Autodesk Fusion 360 part; units mm, degrees
(part 3 of 5)
  line L423 (12.6531, -24.0922) -> (12.4457, -24.1094)
  line L424 (12.4457, -24.1094) -> (12.4457, -24.8166)
  line L425 (12.4457, -24.8166) -> (12.4457, -25.5237)
  line L426 (12.4457, -25.5237) -> (12.7147, -25.4972)
  spline S462 degree 3 poles (12.7147, -25.4972) (13.8566, -25.3848) (14.5858, -24.55) (14.5858, -23.3547) knots 0 0 0 0 1 1 1 1
  spline S463 degree 3 poles (14.5858, -23.3547) (14.5858, -21.5094) (12.6861, -20.5298) (11.4358, -21.7302) knots 0 0 0 0 1 1 1 1
  spline S464 degree 3 poles (11.4358, -21.7302) (11.2215, -21.9362) (11.1899, -21.9548) (11.1445, -21.9001) knots 0 0 0 0 1 1 1 1
  spline S465 degree 3 poles (11.1445, -21.9001) (10.8088, -21.4956) (9.9864, -21.3436) (9.4539, -21.5878) knots 0 0 0 0 1 1 1 1
  spline S466 degree 3 poles (9.4539, -21.5878) (8.7681, -21.9022) (8.3471, -22.7631) (8.4716, -23.5972) knots 0 0 0 0 1 1 1 1
  spline S467 degree 3 poles (8.8609, -38.3358) (9.1911, -37.3218) (10.383, -36.7997) (11.3154, -37.2606) knots 0 0 0 0 1 1 1 1
  spline S468 degree 3 poles (11.3154, -37.2606) (11.5789, -37.391) (11.712, -37.5031) (12.4391, -38.2065) knots 0 0 0 0 1 1 1 1
  spline S469 degree 3 poles (12.4391, -38.2065) (13.0246, -38.7727) (13.2898, -39.0048) (13.352, -39.0048) knots 0 0 0 0 1 1 1 1
  line L427 (13.352, -39.0048) -> (13.4394, -39.0048)
  line L428 (13.4394, -39.0048) -> (13.4394, -38.0493)
  line L429 (13.4394, -38.0493) -> (13.4394, -37.0938)
  line L430 (13.4394, -37.0938) -> (13.7641, -37.0938)
  line L431 (13.7641, -37.0938) -> (14.0891, -37.0938)
  line L432 (14.0891, -37.0938) -> (14.0888, -38.957)
  line L433 (14.0888, -38.957) -> (14.0888, -40.8199)
  line L434 (14.0888, -40.8199) -> (13.1993, -39.9218)
  spline S470 degree 3 poles (13.1993, -39.9218) (12.7098, -39.4279) (12.0642, -38.7689) (11.7643, -38.4573) knots 0 0 0 0 1 1 1 1
  spline S471 degree 3 poles (11.7643, -38.4573) (11.0509, -37.7164) (10.6839, -37.5864) (10.1068, -37.8698) knots 0 0 0 0 1 1 1 1
  spline S472 degree 3 poles (10.1068, -37.8698) (9.2919, -38.2698) (9.2967, -39.5565) (10.115, -39.9796) knots 0 0 0 0 1 1 1 1
  spline S473 degree 3 poles (10.115, -39.9796) (10.2289, -40.0384) (10.2292, -40.0391) (10.2292, -40.3858) knots 0 0 0 0 1 1 1 1
  line L435 (10.2292, -40.3858) -> (10.2292, -40.7329)
  line L436 (10.2292, -40.7329) -> (10.124, -40.7081)
  spline S474 degree 3 poles (10.124, -40.7081) (9.1475, -40.4787) (8.5366, -39.3316) (8.8609, -38.3358) knots 0 0 0 0 1 1 1 1
  spline S475 degree 3 poles (8.7977, -33.2545) (8.8953, -32.4941) (9.4553, -31.8405) (10.2653, -31.5409) knots 0 0 0 0 1 1 1 1
  spline S476 degree 3 poles (10.2653, -31.5409) (10.5632, -31.4309) (12.2025, -31.3968) (12.6135, -31.4924) knots 0 0 0 0 1 1 1 1
  spline S477 degree 3 poles (12.6135, -31.4924) (14.8462, -32.0115) (14.8204, -35.2664) (12.5795, -35.7369) knots 0 0 0 0 1 1 1 1
  spline S478 degree 3 poles (12.5795, -35.7369) (12.2114, -35.8143) (10.8463, -35.8146) (10.4824, -35.7376) knots 0 0 0 0 1 1 1 1
  spline S479 degree 3 poles (10.4824, -35.7376) (9.5743, -35.545) (8.8991, -34.8178) (8.7787, -33.9026) knots 0 0 0 0 1 1 1 1
  spline S480 degree 3 poles (8.7787, -33.9026) (8.7488, -33.6759) (8.7505, -33.624) (8.7977, -33.2545) knots 0 0 0 0 1 1 1 1
  spline S481 degree 3 poles (8.8609, -27.5968) (9.1953, -26.5704) (10.3726, -26.0555) (11.3178, -26.5226) knots 0 0 0 0 1 1 1 1
  spline S482 degree 3 poles (11.3178, -26.5226) (11.5782, -26.6516) (11.7144, -26.7661) (12.4391, -27.4674) knots 0 0 0 0 1 1 1 1
  spline S483 degree 3 poles (12.4391, -27.4674) (13.0246, -28.0336) (13.2898, -28.2654) (13.352, -28.2654) knots 0 0 0 0 1 1 1 1
  line L437 (13.352, -28.2654) -> (13.4394, -28.2654)
  line L438 (13.4394, -28.2654) -> (13.4394, -27.3103)
  line L439 (13.4394, -27.3103) -> (13.4394, -26.3547)
  line L440 (13.4394, -26.3547) -> (13.7641, -26.3547)
  line L441 (13.7641, -26.3547) -> (14.0891, -26.3547)
  line L442 (14.0891, -26.3547) -> (14.0888, -28.218)
  line L443 (14.0888, -28.218) -> (14.0888, -30.0808)
  line L444 (14.0888, -30.0808) -> (13.2182, -29.202)
  spline S484 degree 3 poles (13.2182, -29.202) (12.7398, -28.7184) (12.0938, -28.0594) (11.7829, -27.7371) knots 0 0 0 0 1 1 1 1
  spline S485 degree 3 poles (11.7829, -27.7371) (11.0485, -26.9756) (10.6881, -26.8452) (10.1068, -27.1307) knots 0 0 0 0 1 1 1 1
  spline S486 degree 3 poles (10.1068, -27.1307) (9.2919, -27.5304) (9.2967, -28.8175) (10.115, -29.2406) knots 0 0 0 0 1 1 1 1
  spline S487 degree 3 poles (10.115, -29.2406) (10.2289, -29.2994) (10.2292, -29.2997) (10.2292, -29.6464) knots 0 0 0 0 1 1 1 1
  line L445 (10.2292, -29.6464) -> (10.2292, -29.9938)
  line L446 (10.2292, -29.9938) -> (10.124, -29.9691)
  spline S488 degree 3 poles (10.124, -29.9691) (9.1502, -29.7417) (8.5373, -28.5905) (8.8609, -27.5968) knots 0 0 0 0 1 1 1 1
  spline S489 degree 3 poles (8.8541, -22.7748) (9.1798, -21.8238) (10.3131, -21.5345) (10.9852, -22.231) knots 0 0 0 0 1 1 1 1
  spline S490 degree 3 poles (10.9852, -22.231) (11.2074, -22.4611) (11.2642, -22.4635) (11.4121, -22.2486) knots 0 0 0 0 1 1 1 1
  spline S491 degree 3 poles (11.4121, -22.2486) (12.1451, -21.1833) (13.8064, -21.5142) (14.2081, -22.8051) knots 0 0 0 0 1 1 1 1
  spline S492 degree 3 poles (14.2081, -22.8051) (14.5301, -23.8397) (13.9237, -24.8733) (12.855, -25.1103) knots 0 0 0 0 1 1 1 1
  line L447 (12.855, -25.1103) -> (12.7484, -25.134)
  line L448 (12.7484, -25.134) -> (12.7594, -24.8007)
  line L449 (12.7594, -24.8007) -> (12.7707, -24.4674)
  line L450 (12.7707, -24.4674) -> (12.9007, -24.4341)
  spline S493 degree 3 poles (12.9007, -24.4341) (13.6213, -24.2476) (13.858, -23.0627) (13.288, -22.4928) knots 0 0 0 0 1 1 1 1
  spline S494 degree 3 poles (13.288, -22.4928) (12.7181, -21.9228) (11.8173, -22.284) (11.7313, -23.1174) knots 0 0 0 0 1 1 1 1
  line L451 (11.7313, -23.1174) -> (11.7089, -23.3355)
  line L452 (11.7089, -23.3355) -> (11.354, -23.3355)
  line L453 (11.354, -23.3355) -> (10.999, -23.3355)
  line L454 (10.999, -23.3355) -> (10.9546, -23.1229)
  spline S495 degree 3 poles (10.9546, -23.1229) (10.7974, -22.3645) (9.6995, -22.3026) (9.4997, -23.041) knots 0 0 0 0 1 1 1 1
  spline S496 degree 3 poles (9.4997, -23.041) (9.3924, -23.4376) (9.5282, -23.8304) (9.8275, -23.9893) knots 0 0 0 0 1 1 1 1
  line L455 (9.8275, -23.9893) -> (9.9998, -24.0805)
  line L456 (9.9998, -24.0805) -> (9.9998, -24.4193)
  line L457 (9.9998, -24.4193) -> (9.9998, -24.7577)
  line L458 (9.9998, -24.7577) -> (9.8945, -24.7323)
  spline S497 degree 3 poles (9.8945, -24.7323) (9.0415, -24.5238) (8.5634, -23.6244) (8.8541, -22.7748) knots 0 0 0 0 1 1 1 1
  spline S498 degree 3 poles (9.5551, -34.1155) (9.661, -34.5079) (9.9492, -34.8419) (10.3393, -35.0249) knots 0 0 0 0 1 1 1 1
  line L459 (10.3393, -35.0249) -> (10.5539, -35.1257)
  line L460 (10.5539, -35.1257) -> (11.5476, -35.1257)
  spline S499 degree 3 poles (11.5476, -35.1257) (12.4914, -35.1257) (12.5502, -35.1215) (12.7215, -35.0414) knots 0 0 0 0 1 1 1 1
  spline S500 degree 3 poles (12.7215, -35.0414) (13.9292, -34.4783) (13.8026, -32.5095) (12.5351, -32.1412) knots 0 0 0 0 1 1 1 1
  spline S501 degree 3 poles (12.5351, -32.1412) (12.2001, -32.0438) (10.6189, -32.0792) (10.3819, -32.1896) knots 0 0 0 0 1 1 1 1
  spline S502 degree 3 poles (10.3819, -32.1896) (9.6772, -32.5181) (9.3377, -33.3089) (9.5551, -34.1155) knots 0 0 0 0 1 1 1 1
  spline S503 degree 3 poles (9.8687, -33.2236) (9.952, -32.9801) (10.189, -32.7242) (10.4504, -32.5959) knots 0 0 0 0 1 1 1 1
  line L461 (10.4504, -32.5959) -> (10.6684, -32.4885)
  line L462 (10.6684, -32.4885) -> (11.5283, -32.4885)
  spline S504 degree 3 poles (11.5283, -32.4885) (12.3528, -32.4885) (12.3968, -32.4923) (12.5901, -32.5797) knots 0 0 0 0 1 1 1 1
  spline S505 degree 3 poles (12.5901, -32.5797) (13.4579, -32.9718) (13.4652, -34.263) (12.6018, -34.6624) knots 0 0 0 0 1 1 1 1
  spline S506 degree 3 poles (12.6018, -34.6624) (12.3528, -34.7776) (10.9175, -34.8058) (10.5869, -34.7019) knots 0 0 0 0 1 1 1 1
  spline S507 degree 3 poles (10.5869, -34.7019) (9.9853, -34.5127) (9.6589, -33.8403) (9.8687, -33.2236) knots 0 0 0 0 1 1 1 1
  spline S508 degree 3 poles (10.0792, -95.4233) (10.1329, -95.5155) (10.3296, -95.5117) (10.3802, -95.4174) knots 0 0 0 0 1 1 1 1
  spline S509 degree 3 poles (10.3802, -95.4174) (10.428, -95.3277) (13.039, -45.5861) (13.0029, -45.4434) knots 0 0 0 0 1 1 1 1
  spline S510 degree 3 poles (13.0029, -45.4434) (12.9891, -45.3877) (12.9362, -45.3006) (12.8853, -45.2501) knots 0 0 0 0 1 1 1 1
  line L463 (12.8853, -45.2501) -> (12.7931, -45.1579)
  line L464 (12.7931, -45.1579) -> (11.5469, -45.1579)
  spline S511 degree 3 poles (11.5469, -45.1579) (10.221, -45.1579) (10.1921, -45.1617) (10.0958, -45.3481) knots 0 0 0 0 1 1 1 1
  spline S512 degree 3 poles (10.0958, -45.3481) (10.0246, -45.4857) (10.008, -95.3012) (10.0792, -95.4233) knots 0 0 0 0 1 1 1 1
  spline S513 degree 3 poles (10.0975, -17.0765) (10.1941, -17.2543) (10.2306, -17.2588) (11.5469, -17.2588) knots 0 0 0 0 1 1 1 1
  line L465 (11.5469, -17.2588) -> (12.7931, -17.2588)
  line L466 (12.7931, -17.2588) -> (12.8853, -17.1666)
  spline S514 degree 3 poles (12.8853, -17.1666) (12.9362, -17.116) (12.9891, -17.029) (13.0029, -16.9733) knots 0 0 0 0 1 1 1 1
  spline S515 degree 3 poles (13.0029, -16.9733) (13.039, -16.8305) (10.428, 32.911) (10.3802, 33.0008) knots 0 0 0 0 1 1 1 1
  spline S516 degree 3 poles (10.3802, 33.0008) (10.3272, 33.0995) (10.1305, 33.0988) (10.0775, 32.9997) knots 0 0 0 0 1 1 1 1
  spline S517 degree 3 poles (10.0775, 32.9997) (10.007, 32.8677) (10.027, -16.9461) (10.0975, -17.0765) knots 0 0 0 0 1 1 1 1
extrude "Extrude28" add sketch "Sketch16" along normal blind 3.175 contours S328 S329 S330 | S331 L193 L194 L195 L196 S332 S333 S334 L197 L198 L199 L200 S335 S336 | S337 S338 S339 | S364 S365 S366 S367 L215 L216 L217 L218 L219 L220 | S368 S369 S370 S371 S372 S373 L221 L222 L223 L224 L225 L226 L227 L228 L229 L230 L231 L232 S374 | L233 L234 L235 L236 L237 L238 L239 L240 L241 L242 L243 L244 L245 L246 L247 L248 L249 L250 L251 L252 L253 L254 L255 L256 | L257 L258 L259 L260 L261 L262 L263 L264 L265 L266 L267 L268 L269 L270 L271 L272 L273 L274 L275 L276 L277 L278 L279 L280
extrude "Extrude29" add sketch "Sketch16" along normal blind 1.5875 contours S262 S263 S264 S265 | S266 S267 S268 S269 L73 L74 S270 S271 L75 L76 S272 L77 L78 S273 S274 | S275 S276 S277 S278 | L93 L94 S306 S307 L95 L96 S308 S309 L97 L98 | L99 L100 L101 L102 L103 L104 L105 L106 S310 S311 S312 S313 S314 S315 S316 L107 L108 | L109 L110 L111 L112 L113 L114 L115 L116 L117 L118 L119 L120 L121 L122 L123 L124 L125 L126 L127 L128 | L129 L130 L131 L132 L133 L134 L135 L136 L137 L138 L139 L140 L141 L142 L143 L144 L145 L146 L147 L148 L149 L150 L151 L152
extrude "Extrude30" cut 7 faces at (-0.0754, 98.1019, -3.175) (0.0373, 90.3692, -3.175) (4.1954, 77.1885, -3.175) (0.8786, 64.2283, -3.175) (3.3067, 54.4249, -3.175) (0.2799, 51.1961, -3.175) (4.1954, 36.6395, -3.175) along direction (0, 0, 1) blind 0.7937
sketch "Sketch17" plane through (0, 0, 0) normal (0, 0, -1) x (1, 0, 0)
  spline S0 degree 3 poles (-4.6573, -35.5439) (-2.9984, -31.1371) (3.682, -31.3762) (4.9739, -35.8889) knots -1 -1 -1 -1 0 0 0 0
  spline S1 degree 3 poles (4.9739, -35.8889) (5.9848, -39.4186) (3.6706, -42.6429) (0.1206, -42.6508) knots -1 -1 -1 -1 0 0 0 0
  spline S2 degree 3 poles (0.1206, -42.6508) (-2.4986, -42.6566) (-4.4427, -41.0521) (-4.9222, -38.4889) knots -1 -1 -1 -1 0 0 0 0
  spline S3 degree 3 poles (-4.9222, -38.4889) (-5.0738, -37.6775) (-4.9524, -36.3278) (-4.6573, -35.5439) knots -1 -1 -1 -1 0 0 0 0
  spline S4 degree 3 poles (-4.6573, -76.0925) (-2.9984, -71.6857) (3.682, -71.9251) (4.9739, -76.4378) knots -1 -1 -1 -1 0 0 0 0
  spline S5 degree 3 poles (4.9739, -76.4378) (5.9848, -79.9675) (3.6706, -83.1918) (0.1206, -83.1997) knots -1 -1 -1 -1 0 0 0 0
  spline S6 degree 3 poles (0.1206, -83.1997) (-2.4986, -83.2055) (-4.4427, -81.601) (-4.9222, -79.0378) knots -1 -1 -1 -1 0 0 0 0
  spline S7 degree 3 poles (-4.9222, -79.0378) (-5.0738, -78.2264) (-4.9524, -76.8767) (-4.6573, -76.0925) knots -1 -1 -1 -1 0 0 0 0
  line L0 (-4.6759, -91.3629) -> (-4.6759, -89.0931)
  spline S8 degree 3 poles (-4.6759, -89.0931) (-4.6759, -86.6441) (-4.6683, -86.532) (-4.4654, -85.9352) knots -1 -1 -1 -1 0 0 0 0
  spline S9 degree 3 poles (-4.4654, -85.9352) (-3.9494, -84.418) (-2.3731, -83.6327) (-0.6908, -84.0544) knots -1 -1 -1 -1 0 0 0 0
  spline S10 degree 3 poles (-0.6908, -84.0544) (0.2806, -84.2983) (1.0514, -85.0433) (1.2884, -85.9675) knots -1 -1 -1 -1 0 0 0 0
  spline S11 degree 3 poles (1.2884, -85.9675) (1.3162, -86.0762) (1.3486, -86.165) (1.3602, -86.1646) knots -1 -1 -1 -1 0 0 0 0
  spline S12 degree 3 poles (1.3602, -86.1646) (1.3719, -86.1643) (2.161, -85.5967) (3.1131, -84.9033) knots -1 -1 -1 -1 0 0 0 0
  spline S13 degree 3 poles (3.1131, -84.9033) (4.0655, -84.2102) (4.8611, -83.6427) (4.881, -83.6427) knots -1 -1 -1 -1 0 0 0 0
  spline S14 degree 3 poles (4.881, -83.6427) (4.904, -83.6427) (4.914, -84.1972) (4.9078, -85.1197) knots -1 -1 -1 -1 0 0 0 0
  line L1 (4.9078, -85.1197) -> (4.8979, -86.5963)
  line L2 (4.8979, -86.5963) -> (3.1629, -87.7854)
  line L3 (3.1629, -87.7854) -> (1.428, -88.9741)
  line L4 (1.428, -88.9741) -> (3.1726, -88.984)
  line L5 (3.1726, -88.984) -> (4.9168, -88.994)
  line L6 (4.9168, -88.994) -> (4.9168, -91.3629)
  line L7 (4.9168, -91.3629) -> (-4.6759, -91.3629)
  line L8 (-4.6759, -52.1898) -> (-4.6759, -49.8203)
  line L9 (-4.6759, -49.8203) -> (-0.9305, -49.8203)
  line L10 (-0.9305, -49.8203) -> (-0.9305, -46.1131)
  line L11 (-0.9305, -46.1131) -> (-4.6759, -46.1131)
  line L12 (-4.6759, -46.1131) -> (-4.6759, -43.7821)
  line L13 (-4.6759, -43.7821) -> (4.9168, -43.7821)
  line L14 (4.9168, -43.7821) -> (4.9168, -46.1131)
  line L15 (4.9168, -46.1131) -> (1.0951, -46.1131)
  line L16 (1.0951, -46.1131) -> (1.0951, -49.8203)
  line L17 (1.0951, -49.8203) -> (4.9168, -49.8203)
  line L18 (4.9168, -49.8203) -> (4.9168, -52.1898)
  line L19 (4.9168, -52.1898) -> (-4.6759, -52.1898)
  line L20 (-4.6759, -71.7572) -> (-4.6759, -69.2494)
  line L21 (-4.6759, -69.2494) -> (-1.8964, -67.4364)
  line L22 (-1.8964, -67.4364) -> (0.8832, -65.6234)
  line L23 (0.8832, -65.6234) -> (-1.8964, -65.6135)
  line L24 (-1.8964, -65.6135) -> (-4.6759, -65.6038)
  line L25 (-4.6759, -65.6038) -> (-4.6759, -63.2346)
  line L26 (-4.6759, -63.2346) -> (4.9168, -63.2346)
  line L27 (4.9168, -63.2346) -> (4.9168, -65.7008)
  line L28 (4.9168, -65.7008) -> (2.1183, -67.5348)
  line L29 (2.1183, -67.5348) -> (-0.6805, -69.3684)
  line L30 (-0.6805, -69.3684) -> (2.1183, -69.3784)
  line L31 (2.1183, -69.3784) -> (4.9168, -69.3881)
  line L32 (4.9168, -69.3881) -> (4.9168, -71.7572)
  line L33 (4.9168, -71.7572) -> (-4.6759, -71.7572)
  line L34 (-4.6793, -99.0827) -> (-4.6662, -96.8184)
  spline S15 degree 3 poles (-4.6662, -96.8184) (-4.6521, -94.3474) (-4.6642, -94.4932) (-4.4275, -93.9425) knots -1 -1 -1 -1 0 0 0 0
  spline S16 degree 3 poles (-4.4275, -93.9425) (-3.7197, -92.2936) (-1.5407, -91.8086) (-0.3303, -93.0304) knots -1 -1 -1 -1 0 0 0 0
  line L35 (-0.3303, -93.0304) -> (-0.017, -93.3468)
  line L36 (-0.017, -93.3468) -> (0.1781, -93.1012)
  spline S17 degree 3 poles (0.1781, -93.1012) (1.8174, -91.0416) (4.6598, -91.9245) (4.8783, -94.5617) knots -1 -1 -1 -1 0 0 0 0
  spline S18 degree 3 poles (4.8783, -94.5617) (4.8989, -94.8097) (4.9157, -95.9282) (4.9161, -97.0478) knots -1 -1 -1 -1 0 0 0 0
  line L37 (4.9161, -97.0478) -> (4.9168, -99.0827)
  line L38 (4.9168, -99.0827) -> (-4.6793, -99.0827)
  spline S19 degree 3 poles (-4.8554, -55.553) (-4.6312, -54.613) (-4.1995, -53.8119) (-3.537, -53.1061) knots -1 -1 -1 -1 0 0 0 0
  line L39 (-3.537, -53.1061) -> (-3.2426, -52.7924)
  line L40 (-3.2426, -52.7924) -> (-2.576, -53.4944)
  spline S20 degree 3 poles (-2.576, -53.4944) (-2.2094, -53.8803) (-1.8592, -54.2504) (-1.798, -54.3172) knots -1 -1 -1 -1 0 0 0 0
  line L41 (-1.798, -54.3172) -> (-1.6865, -54.4379)
  line L42 (-1.6865, -54.4379) -> (-1.8757, -54.6656)
  spline S21 degree 3 poles (-1.8757, -54.6656) (-3.6774, -56.8305) (-2.5523, -59.6901) (0.1014, -59.6901) knots -1 -1 -1 -1 0 0 0 0
  spline S22 degree 3 poles (0.1014, -59.6901) (2.7553, -59.6901) (3.8804, -56.8305) (2.0781, -54.6649) knots -1 -1 -1 -1 0 0 0 0
  line L43 (2.0781, -54.6649) -> (1.8882, -54.4365)
  line L44 (1.8882, -54.4365) -> (2.2081, -54.1063)
  spline S23 degree 3 poles (2.2081, -54.1063) (3.1217, -53.1625) (3.4102, -52.8777) (3.4529, -52.8777) knots -1 -1 -1 -1 0 0 0 0
  spline S24 degree 3 poles (3.4529, -52.8777) (3.479, -52.8777) (3.6317, -53.028) (3.7927, -53.212) knots -1 -1 -1 -1 0 0 0 0
  spline S25 degree 3 poles (3.7927, -53.212) (6.5392, -56.3479) (5.118, -61.174) (1.1996, -62.0184) knots -1 -1 -1 -1 0 0 0 0
  spline S26 degree 3 poles (1.1996, -62.0184) (-1.6762, -62.6382) (-4.4138, -60.7987) (-4.9242, -57.9033) knots -1 -1 -1 -1 0 0 0 0
  spline S27 degree 3 poles (-4.9242, -57.9033) (-5.0154, -57.3877) (-4.9762, -56.06) (-4.8554, -55.553) knots -1 -1 -1 -1 0 0 0 0
  circle A0 centre (11.5, 0) radius 2
  circle A1 centre (0, -11.5) radius 2
  circle A2 centre (0, 11.5) radius 2
  circle A3 centre (-11.5, 0) radius 2
  line L45 (-14.4115, 0.4) -> (-14.4075, -127)
  line L46 (-14.4075, -127) -> (14.4182, -127)
  line L47 (14.4182, -127) -> (14.4182, 127.8)
  line L48 (14.4182, 127.8) -> (-14.4075, 127.8)
  line L49 (-14.4075, 127.8) -> (-14.4115, 0.4)
  spline S28 degree 3 poles (-41.1368, 27.9125) (-41.0058, 27.3034) (-40.9336, 27.1434) (-40.2646, 25.9826) knots 0 0 0 0 1 1 1 1
  spline S29 degree 3 poles (-40.2646, 25.9826) (-40.0221, 25.5622) (-39.6654, 24.9431) (-39.4721, 24.6067) knots 0 0 0 0 1 1 1 1
  spline S30 degree 3 poles (-39.4721, 24.6067) (-39.1408, 24.0313) (-37.9129, 21.9022) (-36.7496, 19.8869) knots 0 0 0 0 1 1 1 1
  spline S31 degree 3 poles (-36.7496, 19.8869) (-36.4645, 19.393) (-36.1508, 18.8513) (-36.0521, 18.6831) knots 0 0 0 0 1 1 1 1
  spline S32 degree 3 poles (-36.0521, 18.6831) (-35.9534, 18.5149) (-35.5661, 17.8442) (-35.1915, 17.1927) knots 0 0 0 0 1 1 1 1
  spline S33 degree 3 poles (-35.1915, 17.1927) (-33.8969, 14.9408) (-33.2409, 14.3468) (-31.7334, 14.061) knots 0 0 0 0 1 1 1 1
  spline S34 degree 3 poles (-31.7334, 14.061) (-31.2535, 13.9698) (-18.2743, 13.9708) (-17.8306, 14.062) knots 0 0 0 0 1 1 1 1
  spline S35 degree 3 poles (-17.8306, 14.062) (-16.7915, 14.2753) (-15.8703, 14.8634) (-15.265, 15.7003) knots 0 0 0 0 1 1 1 1
  spline S36 degree 3 poles (-15.265, 15.7003) (-15.1343, 15.8812) (-14.6091, 16.7634) (-14.6242, 16.7769) knots 0 0 0 0 1 1 1 1
  spline S37 degree 3 poles (-14.6242, 16.7769) (-14.6314, 16.7834) (-15.4033, 16.9007) (-15.5443, 16.9168) knots 0 0 0 0 1 1 1 1
  spline S38 degree 3 poles (-15.5443, 16.9168) (-15.5972, 16.923) (-15.6633, 16.8463) (-15.7926, 16.63) knots 0 0 0 0 1 1 1 1
  spline S39 degree 3 poles (-15.7926, 16.63) (-16.2858, 15.8041) (-16.8785, 15.3288) (-17.7659, 15.0467) knots 0 0 0 0 1 1 1 1
  line L50 (-17.7659, 15.0467) -> (-18.1092, 14.9377)
  line L51 (-18.1092, 14.9377) -> (-24.7782, 14.9377)
  line L52 (-24.7782, 14.9377) -> (-31.4472, 14.9377)
  line L53 (-31.4472, 14.9377) -> (-31.7451, 15.024)
  spline S40 degree 3 poles (-31.7451, 15.024) (-32.8681, 15.3498) (-33.2526, 15.7333) (-34.332, 17.6048) knots 0 0 0 0 1 1 1 1
  spline S41 degree 3 poles (-34.332, 17.6048) (-34.7592, 18.345) (-35.1891, 19.0883) (-35.2875, 19.2565) knots 0 0 0 0 1 1 1 1
  spline S42 degree 3 poles (-35.2875, 19.2565) (-35.3862, 19.4246) (-35.6349, 19.8546) (-35.8406, 20.212) knots 0 0 0 0 1 1 1 1
  spline S43 degree 3 poles (-35.8406, 20.212) (-36.0459, 20.569) (-36.2791, 20.9731) (-36.3586, 21.11) knots 0 0 0 0 1 1 1 1
  spline S44 degree 3 poles (-36.3586, 21.11) (-36.4384, 21.2466) (-37.0482, 22.3043) (-37.7141, 23.4603) knots 0 0 0 0 1 1 1 1
  spline S45 degree 3 poles (-37.7141, 23.4603) (-38.38, 24.6164) (-39.0153, 25.717) (-39.1264, 25.9062) knots 0 0 0 0 1 1 1 1
  spline S46 degree 3 poles (-39.1264, 25.9062) (-40.193, 27.7271) (-40.3344, 28.1017) (-40.2835, 28.9685) knots 0 0 0 0 1 1 1 1
  spline S47 degree 3 poles (-40.2835, 28.9685) (-40.2453, 29.6175) (-40.127, 29.926) (-39.4979, 31.0154) knots 0 0 0 0 1 1 1 1
  line L54 (-39.4979, 31.0154) -> (-39.1295, 31.6531)
  line L55 (-39.1295, 31.6531) -> (-39.0865, 31.4549)
  spline S48 degree 3 poles (-39.0865, 31.4549) (-39.0628, 31.3459) (-38.9981, 31.0504) (-38.9431, 30.798) knots 0 0 0 0 1 1 1 1
  spline S49 degree 3 poles (-38.9431, 30.798) (-38.747, 29.9009) (-38.3429, 28.7146) (-37.9968, 28.0205) knots 0 0 0 0 1 1 1 1
  line L56 (-37.9968, 28.0205) -> (-37.8507, 27.7271)
  line L57 (-37.8507, 27.7271) -> (-38.1165, 27.8007)
  spline S50 degree 3 poles (-38.1165, 27.8007) (-38.2631, 27.8413) (-38.3938, 27.8743) (-38.4075, 27.8743) knots 0 0 0 0 1 1 1 1
  spline S51 degree 3 poles (-38.4075, 27.8743) (-38.4213, 27.8743) (-38.423, 27.724) (-38.4113, 27.54) knots 0 0 0 0 1 1 1 1
  spline S52 degree 3 poles (-38.4113, 27.54) (-38.3178, 26.0575) (-36.1488, 23.1838) (-33.8222, 21.4585) knots 0 0 0 0 1 1 1 1
  line L58 (-33.8222, 21.4585) -> (-33.4838, 21.2074)
  line L59 (-33.4838, 21.2074) -> (-33.7073, 21.0182)
  spline S53 degree 3 poles (-33.7073, 21.0182) (-34.925, 19.9884) (-34.938, 19.6974) (-33.7785, 19.4291) knots 0 0 0 0 1 1 1 1
  spline S54 degree 3 poles (-33.7785, 19.4291) (-32.6995, 19.1797) (-32.0536, 19.1935) (-31.4998, 19.4776) knots 0 0 0 0 1 1 1 1
  line L60 (-31.4998, 19.4776) -> (-31.247, 19.6073)
  line L61 (-31.247, 19.6073) -> (-31.0303, 19.4797)
  spline S55 degree 3 poles (-31.0303, 19.4797) (-30.7459, 19.3122) (-30.5013, 19.1295) (-30.0139, 18.7199) knots 0 0 0 0 1 1 1 1
  spline S56 degree 3 poles (-30.0139, 18.7199) (-28.6677, 17.5883) (-26.9489, 17.0637) (-25.5043, 17.3434) knots 0 0 0 0 1 1 1 1
  spline S57 degree 3 poles (-25.5043, 17.3434) (-24.8755, 17.4651) (-20.997, 17.5329) (-19.7719, 17.4431) knots 0 0 0 0 1 1 1 1
  spline S58 degree 3 poles (-19.7719, 17.4431) (-19.4881, 17.4225) (-18.5178, 17.4049) (-17.6159, 17.4042) knots 0 0 0 0 1 1 1 1
  spline S59 degree 3 poles (-17.6159, 17.4042) (-16.0647, 17.4029) (-15.9343, 17.3974) (-15.2082, 17.3014) knots 0 0 0 0 1 1 1 1
  spline S60 degree 3 poles (-15.2082, 17.3014) (-14.1585, 17.1631) (-13.4705, 17.1642) (-12.6822, 17.3052) knots 0 0 0 0 1 1 1 1
  spline S61 degree 3 poles (-12.6822, 17.3052) (-11.4467, 17.5263) (-11.447, 17.5263) (-10.9435, 17.4968) knots 0 0 0 0 1 1 1 1
  spline S62 degree 3 poles (-10.9435, 17.4968) (-10.0489, 17.4445) (-9.9935, 17.4483) (-9.7586, 17.5824) knots 0 0 0 0 1 1 1 1
  spline S63 degree 3 poles (-9.7586, 17.5824) (-9.643, 17.6484) (-9.4376, 17.731) (-9.3018, 17.7657) knots 0 0 0 0 1 1 1 1
  spline S64 degree 3 poles (-9.3018, 17.7657) (-8.7215, 17.9154) (-8.543, 18.1451) (-8.3824, 18.9507) knots 0 0 0 0 1 1 1 1
  spline S65 degree 3 poles (-8.3824, 18.9507) (-8.283, 19.4473) (-8.2771, 19.4604) (-8.0167, 19.7428) knots 0 0 0 0 1 1 1 1
  spline S66 degree 3 poles (-8.0167, 19.7428) (-7.4798, 20.3255) (-7.3873, 21.0313) (-7.7708, 21.6126) knots 0 0 0 0 1 1 1 1
  line L62 (-7.7708, 21.6126) -> (-7.9136, 21.8289)
  line L63 (-7.9136, 21.8289) -> (-7.7564, 21.9861)
  line L64 (-7.7564, 21.9861) -> (-7.5995, 22.1433)
  line L65 (-7.5995, 22.1433) -> (-7.6033, 22.5536)
  spline S67 degree 3 poles (-7.6033, 22.5536) (-7.6085, 23.1294) (-7.6886, 23.3306) (-8.0611, 23.7007) knots 0 0 0 0 1 1 1 1
  spline S68 degree 3 poles (-8.0611, 23.7007) (-8.6661, 24.3023) (-10.0413, 24.6521) (-10.6611, 24.3622) knots 0 0 0 0 1 1 1 1
  spline S69 degree 3 poles (-10.6611, 24.3622) (-11.2603, 24.0815) (-11.7208, 24.2074) (-12.817, 24.951) knots 0 0 0 0 1 1 1 1
  spline S70 degree 3 poles (-12.817, 24.951) (-14.3645, 26.0008) (-15.4459, 26.5092) (-16.6188, 26.7386) knots 0 0 0 0 1 1 1 1
  line L66 (-16.6188, 26.7386) -> (-17.0773, 26.8284)
  line L67 (-17.0773, 26.8284) -> (-17.2304, 27.1052)
  spline S71 degree 3 poles (-17.2304, 27.1052) (-17.792, 28.122) (-19.2869, 29.0558) (-20.8185, 29.3465) knots 0 0 0 0 1 1 1 1
  spline S72 degree 3 poles (-20.8185, 29.3465) (-21.2585, 29.4297) (-21.4256, 29.5821) (-21.9729, 30.3969) knots 0 0 0 0 1 1 1 1
  spline S73 degree 3 poles (-21.9729, 30.3969) (-22.4293, 31.0769) (-22.4795, 31.7287) (-22.1369, 32.5277) knots 0 0 0 0 1 1 1 1
  spline S74 degree 3 poles (-22.1369, 32.5277) (-21.752, 33.4262) (-19.7908, 35.2378) (-18.1078, 36.2497) knots 0 0 0 0 1 1 1 1
  spline S75 degree 3 poles (-18.1078, 36.2497) (-17.4016, 36.6745) (-17.4023, 36.6742) (-15.9691, 36.6852) knots 0 0 0 0 1 1 1 1
  spline S76 degree 3 poles (-15.9691, 36.6852) (-14.8271, 36.6938) (-14.5145, 36.7141) (-13.6167, 36.8396) knots 0 0 0 0 1 1 1 1
  line L68 (-13.6167, 36.8396) -> (-13.4427, 36.864)
  line L69 (-13.4427, 36.864) -> (-13.0378, 36.1624)
  spline S77 degree 3 poles (-13.0378, 36.1624) (-12.8153, 35.7764) (-11.9919, 34.3514) (-11.208, 32.9955) knots 0 0 0 0 1 1 1 1
  spline S78 degree 3 poles (-11.208, 32.9955) (-9.2643, 29.6337) (-9.2952, 29.7011) (-9.2897, 28.8109) knots 0 0 0 0 1 1 1 1
  spline S79 degree 3 poles (-9.2897, 28.8109) (-9.2849, 28.0301) (-9.3812, 27.7522) (-10.0719, 26.5497) knots 0 0 0 0 1 1 1 1
  spline S80 degree 3 poles (-10.0719, 26.5497) (-11.1712, 24.6366) (-11.1041, 24.7649) (-11.0322, 24.712) knots 0 0 0 0 1 1 1 1
  spline S81 degree 3 poles (-11.0322, 24.712) (-10.9318, 24.6384) (-10.8186, 24.6542) (-10.5552, 24.7787) knots 0 0 0 0 1 1 1 1
  spline S82 degree 3 poles (-10.5552, 24.7787) (-10.387, 24.8582) (-10.2542, 24.8936) (-10.1218, 24.8936) knots 0 0 0 0 1 1 1 1
  spline S83 degree 3 poles (-10.1218, 24.8936) (-9.9467, 24.8939) (-9.9247, 24.9042) (-9.859, 25.0178) knots 0 0 0 0 1 1 1 1
  spline S84 degree 3 poles (-9.859, 25.0178) (-9.8194, 25.0862) (-9.6285, 25.4171) (-9.4345, 25.7535) knots 0 0 0 0 1 1 1 1
  spline S85 degree 3 poles (-9.4345, 25.7535) (-9.2406, 26.0895) (-9.0256, 26.4593) (-8.9564, 26.5752) knots 0 0 0 0 1 1 1 1
  spline S86 degree 3 poles (-8.9564, 26.5752) (-8.371, 27.5551) (-8.1915, 28.7628) (-8.4718, 29.8328) knots 0 0 0 0 1 1 1 1
  spline S87 degree 3 poles (-8.4718, 29.8328) (-8.6152, 30.3801) (-8.6837, 30.5142) (-9.8291, 32.4988) knots 0 0 0 0 1 1 1 1
  spline S88 degree 3 poles (-9.8291, 32.4988) (-10.4055, 33.4974) (-10.9806, 34.4948) (-11.1072, 34.7153) knots 0 0 0 0 1 1 1 1
  spline S89 degree 3 poles (-11.1072, 34.7153) (-11.4594, 35.3289) (-11.7074, 35.7585) (-12.0115, 36.2824) knots 0 0 0 0 1 1 1 1
  spline S90 degree 3 poles (-12.0115, 36.2824) (-12.1642, 36.5452) (-12.5904, 37.2847) (-12.9587, 37.9258) knots 0 0 0 0 1 1 1 1
  spline S91 degree 3 poles (-12.9587, 37.9258) (-13.3271, 38.5666) (-13.7096, 39.2287) (-13.809, 39.3969) knots 0 0 0 0 1 1 1 1
  spline S92 degree 3 poles (-13.809, 39.3969) (-13.9084, 39.5651) (-14.2369, 40.1327) (-14.5392, 40.6582) knots 0 0 0 0 1 1 1 1
  spline S93 degree 3 poles (-14.5392, 40.6582) (-15.6815, 42.6446) (-16.41, 43.2606) (-17.931, 43.5258) knots 0 0 0 0 1 1 1 1
  spline S94 degree 3 poles (-17.931, 43.5258) (-18.4139, 43.6101) (-31.0671, 43.6101) (-31.5473, 43.5258) knots 0 0 0 0 1 1 1 1
  spline S95 degree 3 poles (-31.5473, 43.5258) (-32.627, 43.3363) (-33.6389, 42.7254) (-34.2707, 41.8813) knots 0 0 0 0 1 1 1 1
  spline S96 degree 3 poles (-34.2707, 41.8813) (-34.5019, 41.5728) (-34.6157, 41.3836) (-35.5269, 39.7983) knots 0 0 0 0 1 1 1 1
  spline S97 degree 3 poles (-35.5269, 39.7983) (-36.1553, 38.7056) (-36.4769, 38.1477) (-37.5989, 36.206) knots 0 0 0 0 1 1 1 1
  spline S98 degree 3 poles (-37.5989, 36.206) (-37.8479, 35.7751) (-38.2008, 35.1645) (-38.3828, 34.8491) knots 0 0 0 0 1 1 1 1
  spline S99 degree 3 poles (-38.3828, 34.8491) (-38.5647, 34.5337) (-38.8829, 33.9834) (-39.0896, 33.6263) knots 0 0 0 0 1 1 1 1
  spline S100 degree 3 poles (-39.0896, 33.6263) (-41.0027, 30.3216) (-41.0209, 30.2855) (-41.1523, 29.5945) knots 0 0 0 0 1 1 1 1
  spline S101 degree 3 poles (-41.1523, 29.5945) (-41.2349, 29.1587) (-41.2273, 28.3345) (-41.1368, 27.9125) knots 0 0 0 0 1 1 1 1
  line L70 (-38.5692, 32.6361) -> (-38.4491, 32.8342)
  line L71 (-38.4491, 32.8342) -> (-38.1967, 32.6712)
  spline S102 degree 3 poles (-38.1967, 32.6712) (-37.593, 32.2818) (-36.4016, 31.791) (-35.7848, 31.6778) knots 0 0 0 0 1 1 1 1
  line L72 (-35.7848, 31.6778) -> (-35.651, 31.6531)
  line L73 (-35.651, 31.6531) -> (-35.6631, 31.2265)
  spline S103 degree 3 poles (-35.6631, 31.2265) (-35.6971, 30.0334) (-35.5964, 29.2773) (-35.2686, 28.2623) knots 0 0 0 0 1 1 1 1
  spline S104 degree 3 poles (-35.2686, 28.2623) (-35.1712, 27.961) (-35.0976, 27.7082) (-35.1052, 27.7006) knots 0 0 0 0 1 1 1 1
  spline S105 degree 3 poles (-35.1052, 27.7006) (-35.1809, 27.625) (-37.0764, 27.583) (-37.1703, 27.6545) knots 0 0 0 0 1 1 1 1
  spline S106 degree 3 poles (-37.1703, 27.6545) (-37.4702, 27.8843) (-38.1908, 29.8101) (-38.4749, 31.1419) knots 0 0 0 0 1 1 1 1
  spline S107 degree 3 poles (-38.4749, 31.1419) (-38.7188, 32.2849) (-38.725, 32.3791) (-38.5692, 32.6361) knots 0 0 0 0 1 1 1 1
  spline S108 degree 3 poles (-37.8527, 33.8723) (-37.7705, 34.0102) (-37.3818, 34.682) (-36.9884, 35.3651) knots 0 0 0 0 1 1 1 1
  spline S109 degree 3 poles (-36.9884, 35.3651) (-36.5952, 36.0482) (-36.0741, 36.9517) (-35.8306, 37.3731) knots 0 0 0 0 1 1 1 1
  line L74 (-35.8306, 37.3731) -> (-35.3876, 38.1387)
  line L75 (-35.3876, 38.1387) -> (-35.0952, 37.9465)
  line L76 (-35.0952, 37.9465) -> (-34.8028, 37.7538)
  line L77 (-34.8028, 37.7538) -> (-34.8923, 37.4673)
  spline S110 degree 3 poles (-34.8923, 37.4673) (-35.1038, 36.788) (-35.3484, 35.073) (-35.5609, 32.7757) knots 0 0 0 0 1 1 1 1
  spline S111 degree 3 poles (-35.5609, 32.7757) (-35.616, 32.1807) (-35.5403, 32.2206) (-36.2657, 32.4046) knots 0 0 0 0 1 1 1 1
  spline S112 degree 3 poles (-36.2657, 32.4046) (-37.3887, 32.6897) (-37.7368, 32.8074) (-37.7805, 32.9157) knots 0 0 0 0 1 1 1 1
  spline S113 degree 3 poles (-37.7805, 32.9157) (-37.8152, 33.0017) (-37.9917, 33.5582) (-37.9989, 33.6047) knots 0 0 0 0 1 1 1 1
  spline S114 degree 3 poles (-37.9989, 33.6047) (-38.0003, 33.614) (-37.9346, 33.7343) (-37.8527, 33.8723) knots 0 0 0 0 1 1 1 1
  spline S115 degree 3 poles (-37.82, 27.4747) (-37.3131, 27.2796) (-36.222, 27.1101) (-35.4722, 27.1101) knots 0 0 0 0 1 1 1 1
  line L78 (-35.4722, 27.1101) -> (-34.8868, 27.1097)
  line L79 (-34.8868, 27.1097) -> (-34.7585, 26.7372)
  spline S116 degree 3 poles (-34.7585, 26.7372) (-34.3313, 25.4979) (-33.7507, 24.2246) (-32.7191, 22.264) knots 0 0 0 0 1 1 1 1
  spline S117 degree 3 poles (-32.7191, 22.264) (-32.5719, 21.984) (-32.4577, 21.7502) (-32.4653, 21.7436) knots 0 0 0 0 1 1 1 1
  spline S118 degree 3 poles (-32.4653, 21.7436) (-32.4729, 21.7374) (-32.6067, 21.6941) (-32.7625, 21.6473) knots 0 0 0 0 1 1 1 1
  line L80 (-32.7625, 21.6473) -> (-33.0459, 21.5623)
  line L81 (-33.0459, 21.5623) -> (-33.2784, 21.7247)
  spline S119 degree 3 poles (-33.2784, 21.7247) (-34.1366, 22.3239) (-35.5035, 23.6061) (-36.177, 24.444) knots 0 0 0 0 1 1 1 1
  spline S120 degree 3 poles (-36.177, 24.444) (-37.1125, 25.608) (-38.2046, 27.6229) (-37.82, 27.4747) knots 0 0 0 0 1 1 1 1
  spline S121 degree 3 poles (-36.2846, 31.0054) (-36.0641, 30.7849) (-35.7291, 30.9225) (-35.7291, 31.2334) knots 0 0 0 0 1 1 1 1
  spline S122 degree 3 poles (-35.7291, 31.2334) (-35.7291, 31.4463) (-35.8437, 31.5609) (-36.0566, 31.5609) knots 0 0 0 0 1 1 1 1
  spline S123 degree 3 poles (-36.0566, 31.5609) (-36.3675, 31.5609) (-36.5051, 31.2259) (-36.2846, 31.0054) knots 0 0 0 0 1 1 1 1
  spline S124 degree 3 poles (-35.5781, 37.2183) (-35.4498, 37.0903) (-35.3202, 37.0659) (-35.163, 37.1406) knots 0 0 0 0 1 1 1 1
  spline S125 degree 3 poles (-35.163, 37.1406) (-34.7612, 37.3311) (-34.9676, 37.9114) (-35.4058, 37.8237) knots 0 0 0 0 1 1 1 1
  spline S126 degree 3 poles (-35.4058, 37.8237) (-35.6596, 37.7731) (-35.7642, 37.4047) (-35.5781, 37.2183) knots 0 0 0 0 1 1 1 1
  spline S127 degree 3 poles (-35.4357, 26.4091) (-35.4134, 26.3702) (-35.336, 26.3138) (-35.2637, 26.2839) knots 0 0 0 0 1 1 1 1
  spline S128 degree 3 poles (-35.2637, 26.2839) (-34.9033, 26.1332) (-34.6298, 26.6337) (-34.9501, 26.8579) knots 0 0 0 0 1 1 1 1
  spline S129 degree 3 poles (-34.9501, 26.8579) (-35.2428, 27.0629) (-35.6156, 26.7183) (-35.4357, 26.4091) knots 0 0 0 0 1 1 1 1
  spline S130 degree 3 poles (-34.9848, 33.2249) (-34.6825, 36.0929) (-34.5913, 36.6449) (-34.2422, 37.717) knots 0 0 0 0 1 1 1 1
  spline S131 degree 3 poles (-34.2422, 37.717) (-34.1053, 38.1367) (-33.9244, 38.7121) (-33.8394, 38.9959) knots 0 0 0 0 1 1 1 1
  spline S132 degree 3 poles (-33.8394, 38.9959) (-33.6248, 39.7148) (-32.9733, 41.675) (-32.8911, 41.8507) knots 0 0 0 0 1 1 1 1
  spline S133 degree 3 poles (-32.8911, 41.8507) (-32.7498, 42.1514) (-31.8799, 42.5445) (-31.1761, 42.625) knots 0 0 0 0 1 1 1 1
  spline S134 degree 3 poles (-31.1761, 42.625) (-30.9705, 42.6487) (-29.5334, 42.6642) (-27.546, 42.6642) knots 0 0 0 0 1 1 1 1
  line L82 (-27.546, 42.6642) -> (-24.2564, 42.6645)
  line L83 (-24.2564, 42.6645) -> (-24.8934, 42.0055)
  spline S135 degree 3 poles (-24.8934, 42.0055) (-25.7134, 41.1563) (-25.9239, 40.9179) (-26.1268, 40.607) knots 0 0 0 0 1 1 1 1
  spline S136 degree 3 poles (-26.1268, 40.607) (-26.9523, 39.3405) (-27.9385, 36.4819) (-28.6525, 33.2824) knots 0 0 0 0 1 1 1 1
  spline S137 degree 3 poles (-28.6525, 33.2824) (-28.8018, 32.6124) (-28.9958, 31.468) (-28.9652, 31.437) knots 0 0 0 0 1 1 1 1
  spline S138 degree 3 poles (-28.9652, 31.437) (-28.9418, 31.4137) (-28.9415, 31.4147) (-28.7736, 31.9551) knots 0 0 0 0 1 1 1 1
  spline S139 degree 3 poles (-28.7736, 31.9551) (-28.1304, 34.025) (-26.3528, 37.7889) (-25.3798, 39.1421) knots 0 0 0 0 1 1 1 1
  spline S140 degree 3 poles (-25.3798, 39.1421) (-24.8876, 39.8265) (-23.9905, 40.5698) (-22.1221, 41.8414) knots 0 0 0 0 1 1 1 1
  spline S141 degree 3 poles (-22.1221, 41.8414) (-21.8487, 42.0275) (-21.4824, 42.2903) (-21.308, 42.4258) knots 0 0 0 0 1 1 1 1
  line L84 (-21.308, 42.4258) -> (-20.9909, 42.6718)
  line L85 (-20.9909, 42.6718) -> (-19.5882, 42.6546)
  spline S142 degree 3 poles (-19.5882, 42.6546) (-17.1609, 42.625) (-16.5999, 42.3302) (-15.5659, 40.5437) knots 0 0 0 0 1 1 1 1
  spline S143 degree 3 poles (-15.5659, 40.5437) (-14.4006, 38.5298) (-13.8929, 37.6403) (-13.9029, 37.6293) knots 0 0 0 0 1 1 1 1
  spline S144 degree 3 poles (-13.9029, 37.6293) (-13.9676, 37.5595) (-15.2653, 37.4271) (-16.2367, 37.391) knots 0 0 0 0 1 1 1 1
  spline S145 degree 3 poles (-16.2367, 37.391) (-17.692, 37.337) (-18.1222, 37.1502) (-19.6976, 35.8868) knots 0 0 0 0 1 1 1 1
  line L86 (-19.6976, 35.8868) -> (-20.1014, 35.5632)
  line L87 (-20.1014, 35.5632) -> (-20.4237, 35.601)
  spline S146 degree 3 poles (-20.4237, 35.601) (-21.7672, 35.7585) (-23.2586, 35.2378) (-24.1749, 34.2912) knots 0 0 0 0 1 1 1 1
  spline S147 degree 3 poles (-24.1749, 34.2912) (-24.9863, 33.4533) (-26.2792, 31.3848) (-26.7401, 30.1868) knots 0 0 0 0 1 1 1 1
  spline S148 degree 3 poles (-26.7401, 30.1868) (-27.1666, 29.0782) (-27.836, 26.893) (-28.1056, 25.728) knots 0 0 0 0 1 1 1 1
  spline S149 degree 3 poles (-28.1056, 25.728) (-28.2363, 25.1646) (-28.2322, 25.1994) (-28.1651, 25.1994) knots 0 0 0 0 1 1 1 1
  spline S150 degree 3 poles (-28.1651, 25.1994) (-28.1311, 25.1994) (-28.0248, 25.457) (-27.8625, 25.9347) knots 0 0 0 0 1 1 1 1
  spline S151 degree 3 poles (-27.8625, 25.9347) (-27.7245, 26.3396) (-27.4635, 27.0488) (-27.2819, 27.5115) knots 0 0 0 0 1 1 1 1
  spline S152 degree 3 poles (-27.2819, 27.5115) (-26.2187, 30.2208) (-25.9084, 30.8403) (-25.0458, 31.9795) knots 0 0 0 0 1 1 1 1
  spline S153 degree 3 poles (-25.0458, 31.9795) (-23.4281, 34.1155) (-22.5834, 34.7752) (-20.9565, 35.1724) knots 0 0 0 0 1 1 1 1
  spline S154 degree 3 poles (-20.9565, 35.1724) (-20.6947, 35.2364) (-20.4677, 35.2887) (-20.4519, 35.2887) knots 0 0 0 0 1 1 1 1
  spline S155 degree 3 poles (-20.4519, 35.2887) (-20.4357, 35.2887) (-20.6772, 35.0349) (-20.9881, 34.7249) knots 0 0 0 0 1 1 1 1
  spline S156 degree 3 poles (-20.9881, 34.7249) (-22.0224, 33.6931) (-22.4953, 33.0172) (-22.6339, 32.3716) knots 0 0 0 0 1 1 1 1
  spline S157 degree 3 poles (-22.6339, 32.3716) (-22.6972, 32.0782) (-22.7065, 32.0613) (-22.8207, 32.0318) knots 0 0 0 0 1 1 1 1
  spline S158 degree 3 poles (-22.8207, 32.0318) (-23.1791, 31.9389) (-24.0576, 30.7956) (-24.3747, 30.0093) knots 0 0 0 0 1 1 1 1
  spline S159 degree 3 poles (-24.3747, 30.0093) (-24.5195, 29.6502) (-24.8652, 28.6056) (-24.9361, 28.3139) knots 0 0 0 0 1 1 1 1
  spline S160 degree 3 poles (-24.9361, 28.3139) (-24.9722, 28.1643) (-25.0365, 28.0635) (-25.2336, 27.8489) knots 0 0 0 0 1 1 1 1
  spline S161 degree 3 poles (-25.2336, 27.8489) (-25.5724, 27.4798) (-26.1943, 26.4603) (-26.0804, 26.4603) knots 0 0 0 0 1 1 1 1
  spline S162 degree 3 poles (-26.0804, 26.4603) (-26.0629, 26.4603) (-25.9789, 26.5508) (-25.8936, 26.6612) knots 0 0 0 0 1 1 1 1
  spline S163 degree 3 poles (-25.8936, 26.6612) (-24.5804, 28.3617) (-22.4905, 29.0754) (-20.5613, 28.4824) knots 0 0 0 0 1 1 1 1
  spline S164 degree 3 poles (-20.5613, 28.4824) (-17.725, 27.6109) (-16.8733, 26.1301) (-17.5561, 23.256) knots 0 0 0 0 1 1 1 1
  spline S165 degree 3 poles (-17.5561, 23.256) (-17.6548, 22.8405) (-17.6328, 22.8288) (-17.4477, 23.1986) knots 0 0 0 0 1 1 1 1
  spline S166 degree 3 poles (-17.4477, 23.1986) (-16.9868, 24.1176) (-16.7653, 25.1502) (-16.864, 25.9224) knots 0 0 0 0 1 1 1 1
  spline S167 degree 3 poles (-16.864, 25.9224) (-16.9136, 26.3114) (-16.9504, 26.2794) (-16.5524, 26.191) knots 0 0 0 0 1 1 1 1
  spline S168 degree 3 poles (-16.5524, 26.191) (-15.4579, 25.9471) (-14.6737, 25.5622) (-13.1348, 24.5142) knots 0 0 0 0 1 1 1 1
  spline S169 degree 3 poles (-13.1348, 24.5142) (-11.9647, 23.7172) (-11.187, 23.5123) (-10.5239, 23.8259) knots 0 0 0 0 1 1 1 1
  spline S170 degree 3 poles (-10.5239, 23.8259) (-10.2408, 23.9597) (-10.0767, 23.9666) (-9.6151, 23.8631) knots 0 0 0 0 1 1 1 1
  spline S171 degree 3 poles (-9.6151, 23.8631) (-8.6066, 23.6375) (-8.1873, 23.2821) (-8.1254, 22.6008) knots 0 0 0 0 1 1 1 1
  line L88 (-8.1254, 22.6008) -> (-8.1058, 22.382)
  line L89 (-8.1058, 22.382) -> (-8.2843, 22.2455)
  spline S172 degree 3 poles (-8.2843, 22.2455) (-8.3923, 22.1632) (-8.5416, 22.092) (-8.6617, 22.0663) knots 0 0 0 0 1 1 1 1
  spline S173 degree 3 poles (-8.6617, 22.0663) (-8.867, 22.0219) (-10.527, 22.0095) (-10.7103, 22.0511) knots 0 0 0 0 1 1 1 1
  spline S174 degree 3 poles (-10.7103, 22.0511) (-11.1306, 22.1457) (-11.607, 22.329) (-11.8729, 22.4979) knots 0 0 0 0 1 1 1 1
  spline S175 degree 3 poles (-11.8729, 22.4979) (-12.1532, 22.6764) (-12.1663, 22.6837) (-12.1663, 22.662) knots 0 0 0 0 1 1 1 1
  spline S176 degree 3 poles (-12.1663, 22.662) (-12.1663, 22.5653) (-11.5595, 22.1378) (-11.1309, 21.9324) knots 0 0 0 0 1 1 1 1
  spline S177 degree 3 poles (-11.1309, 21.9324) (-10.6948, 21.7233) (-9.1147, 21.4619) (-8.6035, 21.5142) knots 0 0 0 0 1 1 1 1
  line L90 (-8.6035, 21.5142) -> (-8.3586, 21.5393)
  line L91 (-8.3586, 21.5393) -> (-8.2286, 21.3374)
  spline S178 degree 3 poles (-8.2286, 21.3374) (-7.959, 20.9171) (-8.0312, 20.5263) (-8.4625, 20.0696) knots 0 0 0 0 1 1 1 1
  spline S179 degree 3 poles (-8.4625, 20.0696) (-8.587, 19.9375) (-8.7091, 19.7755) (-8.7336, 19.7091) knots 0 0 0 0 1 1 1 1
  line L92 (-8.7336, 19.7091) -> (-8.7776, 19.5887)
  line L93 (-8.7776, 19.5887) -> (-8.8584, 19.7088)
  spline S180 degree 3 poles (-8.8584, 19.7088) (-8.9502, 19.845) (-9.1773, 19.9843) (-9.3637, 20.0194) knots 0 0 0 0 1 1 1 1
  spline S181 degree 3 poles (-9.3637, 20.0194) (-10.0227, 20.1432) (-10.9514, 18.7192) (-10.6105, 18.108) knots 0 0 0 0 1 1 1 1
  spline S182 degree 3 poles (-10.6105, 18.108) (-10.5672, 18.0302) (-10.5737, 18.0292) (-11.1275, 18.0251) knots 0 0 0 0 1 1 1 1
  spline S183 degree 3 poles (-11.1275, 18.0251) (-11.5179, 18.022) (-11.8285, 17.9955) (-12.1473, 17.9384) knots 0 0 0 0 1 1 1 1
  spline S184 degree 3 poles (-12.1473, 17.9384) (-12.3995, 17.893) (-12.7606, 17.8283) (-12.9498, 17.7943) knots 0 0 0 0 1 1 1 1
  spline S185 degree 3 poles (-12.9498, 17.7943) (-13.4705, 17.7011) (-14.347, 17.7128) (-15.0328, 17.8221) knots 0 0 0 0 1 1 1 1
  spline S186 degree 3 poles (-15.0328, 17.8221) (-16.1634, 18.0027) (-24.1281, 18.0643) (-25.4279, 17.9023) knots 0 0 0 0 1 1 1 1
  spline S187 degree 3 poles (-25.4279, 17.9023) (-27.0535, 17.7) (-28.4114, 18.0612) (-29.4739, 18.9782) knots 0 0 0 0 1 1 1 1
  spline S188 degree 3 poles (-29.4739, 18.9782) (-30.016, 19.4456) (-30.2698, 19.651) (-30.4535, 19.7696) knots 0 0 0 0 1 1 1 1
  spline S189 degree 3 poles (-30.4535, 19.7696) (-30.5725, 19.8467) (-30.6086, 19.8838) (-30.5491, 19.868) knots 0 0 0 0 1 1 1 1
  spline S190 degree 3 poles (-30.5491, 19.868) (-29.7553, 19.6561) (-29.0924, 20.1198) (-29.2469, 20.7785) knots 0 0 0 0 1 1 1 1
  spline S191 degree 3 poles (-29.2469, 20.7785) (-29.2971, 20.9924) (-29.3153, 20.9852) (-29.3153, 20.751) knots 0 0 0 0 1 1 1 1
  spline S192 degree 3 poles (-29.3153, 20.751) (-29.3153, 20.3812) (-29.5231, 20.17) (-29.9324, 20.1243) knots 0 0 0 0 1 1 1 1
  line L94 (-29.9324, 20.1243) -> (-30.1095, 20.1047)
  line L95 (-30.1095, 20.1047) -> (-29.9847, 20.2099)
  spline S193 degree 3 poles (-29.9847, 20.2099) (-29.024, 21.0206) (-30.0535, 22.1) (-31.6192, 21.9242) knots 0 0 0 0 1 1 1 1
  line L96 (-31.6192, 21.9242) -> (-31.9057, 21.8919)
  line L97 (-31.9057, 21.8919) -> (-32.1444, 22.3321)
  spline S194 degree 3 poles (-32.1444, 22.3321) (-33.417, 24.6786) (-34.0654, 26.2027) (-34.8273, 28.6389) knots 0 0 0 0 1 1 1 1
  spline S195 degree 3 poles (-34.8273, 28.6389) (-35.1798, 29.7654) (-35.2214, 30.9789) (-34.9848, 33.2249) knots 0 0 0 0 1 1 1 1
  spline S196 degree 3 poles (-34.3591, 39.9197) (-34.0826, 40.3965) (-33.8511, 40.7817) (-33.8449, 40.7759) knots 0 0 0 0 1 1 1 1
  spline S197 degree 3 poles (-33.8449, 40.7759) (-33.8391, 40.7697) (-33.9447, 40.4226) (-34.0795, 40.0044) knots 0 0 0 0 1 1 1 1
  spline S198 degree 3 poles (-34.0795, 40.0044) (-34.2143, 39.5865) (-34.3825, 39.0588) (-34.453, 38.8325) knots 0 0 0 0 1 1 1 1
  line L98 (-34.453, 38.8325) -> (-34.581, 38.4204)
  line L99 (-34.581, 38.4204) -> (-34.8194, 38.5621)
  line L100 (-34.8194, 38.5621) -> (-35.0577, 38.7035)
  line L101 (-35.0577, 38.7035) -> (-34.96, 38.8782)
  spline S199 degree 3 poles (-34.96, 38.8782) (-34.9064, 38.9746) (-34.636, 39.443) (-34.3591, 39.9197) knots 0 0 0 0 1 1 1 1
  spline S200 degree 3 poles (-34.1669, 20.1676) (-34.0159, 20.3502) (-33.2526, 21.0478) (-33.0198, 21.216) knots 0 0 0 0 1 1 1 1
  spline S201 degree 3 poles (-33.0198, 21.216) (-32.6913, 21.453) (-31.766, 21.6593) (-31.1414, 21.6349) knots 0 0 0 0 1 1 1 1
  spline S202 degree 3 poles (-31.1414, 21.6349) (-29.6297, 21.5754) (-29.4687, 20.5797) (-30.8931, 20.0974) knots 0 0 0 0 1 1 1 1
  spline S203 degree 3 poles (-30.8931, 20.0974) (-31.0506, 20.0441) (-31.2484, 19.9585) (-31.3326, 19.9076) knots 0 0 0 0 1 1 1 1
  spline S204 degree 3 poles (-31.3326, 19.9076) (-31.8194, 19.6114) (-32.0519, 19.543) (-32.5688, 19.543) knots 0 0 0 0 1 1 1 1
  spline S205 degree 3 poles (-32.5688, 19.543) (-33.1233, 19.543) (-34.4097, 19.8278) (-34.3464, 19.9365) knots 0 0 0 0 1 1 1 1
  spline S206 degree 3 poles (-34.3464, 19.9365) (-34.3316, 19.9619) (-34.2508, 20.0658) (-34.1669, 20.1676) knots 0 0 0 0 1 1 1 1
  spline S207 degree 3 poles (-26.7178, 22.4948) (-26.6706, 22.4508) (-26.5874, 22.3978) (-26.5334, 22.3772) knots 0 0 0 0 1 1 1 1
  spline S208 degree 3 poles (-26.5334, 22.3772) (-26.4371, 22.3407) (-26.4312, 22.316) (-26.2355, 21.1341) knots 0 0 0 0 1 1 1 1
  spline S209 degree 3 poles (-26.2355, 21.1341) (-25.9108, 19.1729) (-25.7017, 18.725) (-25.0176, 18.5259) knots 0 0 0 0 1 1 1 1
  spline S210 degree 3 poles (-25.0176, 18.5259) (-24.5639, 18.3941) (-24.3383, 18.4557) (-23.3449, 18.9823) knots 0 0 0 0 1 1 1 1
  spline S211 degree 3 poles (-23.3449, 18.9823) (-23.0123, 19.1591) (-22.4413, 19.2915) (-21.741, 19.3545) knots 0 0 0 0 1 1 1 1
  line L102 (-21.741, 19.3545) -> (-21.2282, 19.4009)
  line L103 (-21.2282, 19.4009) -> (-21.1271, 19.2809)
  spline S212 degree 3 poles (-21.1271, 19.2809) (-20.9224, 19.0377) (-20.5361, 19.1718) (-20.5361, 19.4855) knots 0 0 0 0 1 1 1 1
  spline S213 degree 3 poles (-20.5361, 19.4855) (-20.5361, 19.6771) (-20.6741, 19.8106) (-20.8715, 19.8106) knots 0 0 0 0 1 1 1 1
  spline S214 degree 3 poles (-20.8715, 19.8106) (-21.0228, 19.8106) (-21.1859, 19.6926) (-21.1859, 19.5836) knots 0 0 0 0 1 1 1 1
  spline S215 degree 3 poles (-21.1859, 19.5836) (-21.1859, 19.5471) (-21.2192, 19.5406) (-21.31, 19.5602) knots 0 0 0 0 1 1 1 1
  spline S216 degree 3 poles (-21.31, 19.5602) (-21.6451, 19.6324) (-22.0186, 19.6603) (-22.5177, 19.6503) knots 0 0 0 0 1 1 1 1
  line L104 (-22.5177, 19.6503) -> (-23.0663, 19.6393)
  line L105 (-23.0663, 19.6393) -> (-23.1554, 19.7511)
  spline S217 degree 3 poles (-23.1554, 19.7511) (-23.2809, 19.9086) (-23.3851, 20.2261) (-23.4574, 20.6705) knots 0 0 0 0 1 1 1 1
  spline S218 degree 3 poles (-23.4574, 20.6705) (-23.5554, 21.2734) (-23.6146, 21.4389) (-23.8048, 21.6422) knots 0 0 0 0 1 1 1 1
  spline S219 degree 3 poles (-23.8048, 21.6422) (-24.34, 22.2145) (-25.3522, 22.23) (-25.8286, 21.6734) knots 0 0 0 0 1 1 1 1
  line L106 (-25.8286, 21.6734) -> (-25.9538, 21.5273)
  line L107 (-25.9538, 21.5273) -> (-26.132, 21.9723)
  spline S220 degree 3 poles (-26.132, 21.9723) (-26.2861, 22.3579) (-26.3026, 22.4236) (-26.2531, 22.4611) knots 0 0 0 0 1 1 1 1
  spline S221 degree 3 poles (-26.2531, 22.4611) (-26.0261, 22.6341) (-26.165, 23.0589) (-26.4484, 23.0589) knots 0 0 0 0 1 1 1 1
  spline S222 degree 3 poles (-26.4484, 23.0589) (-26.7528, 23.0589) (-26.9283, 22.6919) (-26.7178, 22.4948) knots 0 0 0 0 1 1 1 1
  spline S223 degree 3 poles (-26.5527, 22.8078) (-26.4701, 22.8904) (-26.3356, 22.8199) (-26.3525, 22.7029) knots 0 0 0 0 1 1 1 1
  spline S224 degree 3 poles (-26.3525, 22.7029) (-26.3724, 22.5619) (-26.6087, 22.5791) (-26.6122, 22.7218) knots 0 0 0 0 1 1 1 1
  spline S225 degree 3 poles (-26.6122, 22.7218) (-26.6125, 22.7363) (-26.5857, 22.7748) (-26.5527, 22.8078) knots 0 0 0 0 1 1 1 1
  spline S226 degree 3 poles (-25.7818, 21.3247) (-25.3915, 21.777) (-24.9113, 21.8726) (-24.3696, 21.606) knots 0 0 0 0 1 1 1 1
  spline S227 degree 3 poles (-24.3696, 21.606) (-24.1948, 21.52) (-24.1339, 21.4729) (-24.1711, 21.4526) knots 0 0 0 0 1 1 1 1
  spline S228 degree 3 poles (-24.1711, 21.4526) (-24.234, 21.4172) (-25.7664, 20.8528) (-25.8462, 20.8356) knots 0 0 0 0 1 1 1 1
  spline S229 degree 3 poles (-25.8462, 20.8356) (-25.894, 20.8249) (-25.9335, 20.913) (-25.9583, 21.0839) knots 0 0 0 0 1 1 1 1
  spline S230 degree 3 poles (-25.9583, 21.0839) (-25.9611, 21.1011) (-25.8816, 21.2094) (-25.7818, 21.3247) knots 0 0 0 0 1 1 1 1
  spline S231 degree 3 poles (-24.2908, 21.0918) (-23.9709, 21.2091) (-23.9375, 21.2146) (-23.9375, 21.1517) knots 0 0 0 0 1 1 1 1
  spline S232 degree 3 poles (-23.9375, 21.1517) (-23.9375, 21.1049) (-23.9905, 21.0622) (-24.0999, 21.0216) knots 0 0 0 0 1 1 1 1
  spline S233 degree 3 poles (-24.0999, 21.0216) (-24.1893, 20.9883) (-24.503, 20.8734) (-24.7974, 20.7664) knots 0 0 0 0 1 1 1 1
  spline S234 degree 3 poles (-24.7974, 20.7664) (-25.0915, 20.6591) (-25.4355, 20.5312) (-25.5617, 20.4813) knots 0 0 0 0 1 1 1 1
  spline S235 degree 3 poles (-25.5617, 20.4813) (-25.7688, 20.4001) (-25.7932, 20.3974) (-25.8142, 20.4545) knots 0 0 0 0 1 1 1 1
  spline S236 degree 3 poles (-25.8142, 20.4545) (-25.8376, 20.5181) (-25.6852, 20.5817) (-24.2908, 21.0918) knots 0 0 0 0 1 1 1 1
  spline S237 degree 3 poles (-25.2752, 20.3671) (-25.0334, 20.4569) (-24.6224, 20.6099) (-24.362, 20.7066) knots 0 0 0 0 1 1 1 1
  spline S238 degree 3 poles (-24.362, 20.7066) (-24.1016, 20.8036) (-23.8804, 20.8744) (-23.8705, 20.8645) knots 0 0 0 0 1 1 1 1
  spline S239 degree 3 poles (-23.8705, 20.8645) (-23.8605, 20.8545) (-23.8192, 20.6777) (-23.779, 20.4717) knots 0 0 0 0 1 1 1 1
  spline S240 degree 3 poles (-23.779, 20.4717) (-23.6971, 20.0537) (-23.5403, 19.6926) (-23.37, 19.5296) knots 0 0 0 0 1 1 1 1
  line L108 (-23.37, 19.5296) -> (-23.2572, 19.4212)
  line L109 (-23.2572, 19.4212) -> (-23.7638, 19.1615)
  spline S241 degree 3 poles (-23.7638, 19.1615) (-24.8342, 18.6133) (-25.3254, 18.7811) (-25.6625, 19.8106) knots 0 0 0 0 1 1 1 1
  spline S242 degree 3 poles (-25.6625, 19.8106) (-25.7812, 20.1731) (-25.7763, 20.1803) (-25.2752, 20.3671) knots 0 0 0 0 1 1 1 1
  spline S243 degree 3 poles (-24.0641, 29.4414) (-23.8196, 30.1778) (-23.2661, 31.1939) (-22.8984, 31.5815) knots 0 0 0 0 1 1 1 1
  line L110 (-22.8984, 31.5815) -> (-22.7719, 31.7153)
  line L111 (-22.7719, 31.7153) -> (-22.7499, 31.3714)
  spline S244 degree 3 poles (-22.7499, 31.3714) (-22.7175, 30.8671) (-22.4568, 30.3928) (-21.7778, 29.6037) knots 0 0 0 0 1 1 1 1
  line L112 (-21.7778, 29.6037) -> (-21.6382, 29.4414)
  line L113 (-21.6382, 29.4414) -> (-21.8676, 29.4414)
  spline S245 degree 3 poles (-21.8676, 29.4414) (-22.5786, 29.4414) (-23.6538, 29.1188) (-24.1718, 28.7497) knots 0 0 0 0 1 1 1 1
  line L114 (-24.1718, 28.7497) -> (-24.2901, 28.6658)
  line L115 (-24.2901, 28.6658) -> (-24.2626, 28.7955)
  spline S246 degree 3 poles (-24.2626, 28.7955) (-24.2478, 28.867) (-24.1584, 29.1576) (-24.0641, 29.4414) knots 0 0 0 0 1 1 1 1
  spline S247 degree 3 poles (-23.1509, 24.2593) (-21.6967, 21.938) (-19.505, 20.5473) (-18.2798, 21.1682) knots 0 0 0 0 1 1 1 1
  spline S248 degree 3 poles (-18.2798, 21.1682) (-17.8908, 21.3653) (-17.6834, 21.6232) (-18.0232, 21.4874) knots 0 0 0 0 1 1 1 1
  spline S249 degree 3 poles (-18.0232, 21.4874) (-19.0953, 21.0585) (-20.3855, 21.8042) (-23.002, 24.3642) knots 0 0 0 0 1 1 1 1
  spline S250 degree 3 poles (-23.002, 24.3642) (-23.4422, 24.7952) (-23.4732, 24.7735) (-23.1509, 24.2593) knots 0 0 0 0 1 1 1 1